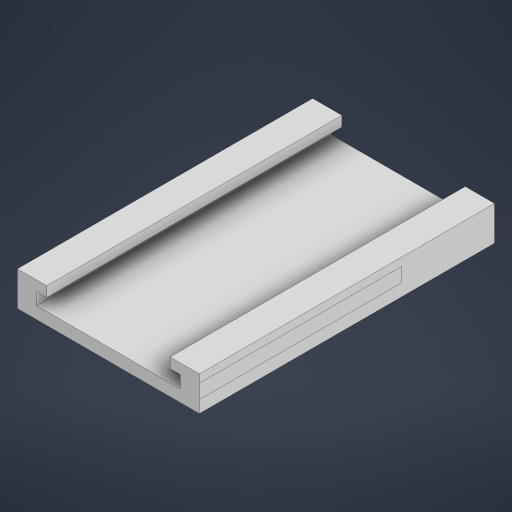
# Autodesk Inventor part: DINsupport
Saved by Autodesk Inventor 2023 (Build 270158000, 158)
## iProperties
Created: 2022-09-20
Part Number: DINsupport
Material: Generic
Document SubType Name: Modeling
Designer: CB110-09
Density: 1 g/cm^3
Appearance: Default
Author: CB110-09
Autodesk Inventor part; units mm, degrees
ref_plane "YZ Plane" through (0, 0, 0) normal (1, 0, 0) x (0, 1, 0)
ref_plane "XZ Plane" through (0, 0, 0) normal (0, 1, 0) x (-1, 0, 0)
ref_plane "XY Plane" through (0, 0, 0) normal (0, 0, 1) x (1, 0, 0)
sketch "Sketch1" plane through (0, 0, 0) normal (0, 1, 0) x (-1, 0, 0)
  line L0 (-32.5, 25) -> (32.5, 25)
  line L1 (32.5, 25) -> (32.5, -25)
  line L2 (32.5, -25) -> (-32.5, -25)
  line L3 (-32.5, -25) -> (-32.5, 25)
  line L4 (-32.5, 25) -> (32.5, -25) construction
  line L5 (32.5, 25) -> (-32.5, -25) construction
  point P0 (0, 0)
  dimension "d0" = 65
  dimension "d1" = 50
  constraints: 12 end point, 2 midpoint, 2 parallel, 1 horizontal, 1 perpendicular
  measures "d0" distance of L1.end L2.end
  measures "d1" distance of L0.end L1.end
extrude "Extrusion1" add sketch "Sketch1" along normal blind 3
sketch "Sketch2" plane through (0, 3, 0) normal (0, 1, 0) x (1, 0, 0)
  line L0 (32.5, 25) -> (-32.5, 25) projected
  line L1 (-18.25, -25) -> (18.25, -25)
  line L2 (18.25, -25) -> (18.25, 25)
  line L3 (18.25, 25) -> (-18.25, 25)
  line L4 (-18.25, 25) -> (-18.25, -25)
  line L5 (-18.25, -25) -> (18.25, 25) construction
  line L6 (18.25, -25) -> (-18.25, 25) construction
  line L7 (-22.5, -25) -> (22.5, -25)
  line L8 (22.5, -25) -> (22.5, 25)
  line L9 (22.5, 25) -> (-22.5, 25)
  line L10 (-22.5, 25) -> (-22.5, -25)
  line L11 (-22.5, -25) -> (22.5, 25) construction
  line L12 (22.5, -25) -> (-22.5, 25) construction
  point P0 (0, 0)
  dimension "d4" = 36.5
  dimension "d5" = 45
  constraints: 24 end point, 4 midpoint, 4 parallel, 2 horizontal, 2 perpendicular, 2 point on line
  measures "d4" distance of L3.end L2.end
  measures "d5" distance of L9.end L8.end
extrude "Extrusion2" add sketch "Sketch2" along normal blind 3.5 contours L8 L7 L2 L0 | L4 L7 L10 L0
sketch "Sketch3" plane through (0, 6.5, 0) normal (0, 1, 0) x (1, 0, 0)
  line L0 (-22.5, 25) -> (-32.5, 25) projected
  line L1 (-22.5, 25) -> (-15.25, 25)
  line L2 (-15.25, 25) -> (-15.25, -25)
  line L3 (-15.25, -25) -> (-22.5, -25)
  line L4 (-22.5, -25) -> (-22.5, 25)
  line L5 (-32.5, -25) -> (32.5, -25) projected
  line L6 (32.5, 25) -> (-32.5, 25) projected
  line L7 (22.4999, -25) -> (15.2499, -25)
  line L8 (15.2499, -25) -> (15.2499, 25)
  line L9 (15.2499, 25) -> (22.4999, 25)
  line L10 (22.4999, 25) -> (22.4999, -25)
  point P0 (0, 0)
  dimension "d8" = 7.25
  dimension "d9" = 7.25
  constraints: 16 end point, 4 parallel, 2 horizontal, 2 perpendicular, 2 point on line
  measures "d8" distance of L2.end L3.end
  measures "d9" distance of L8.end L9.end
extrude "Extrusion3" add sketch "Sketch3" along normal blind 2 contours L1 L2 L3 L4 | L6 L10 L5 L8
sketch "Sketch4" plane through (0, 3, 0) normal (0, 1, 0) x (1, 0, 0)
  line L0 (-22.5, 25) -> (-22.5, -25) projected
  line L1 (-32.5, 25) -> (-32.5, -25) projected
  line L2 (-22.5, 25) -> (-32.5, 25)
  line L3 (-32.5, 25) -> (-32.5, -25)
  line L4 (-32.5, -25) -> (-22.5, -25)
  line L5 (-22.5, -25) -> (-22.5, 25)
  line L6 (22.4999, -25) -> (22.4999, 25) projected
  line L7 (-32.5, -25) -> (32.5, -25) projected
  line L8 (22.4999, 25) -> (32.5, 25)
  line L9 (32.5, 25) -> (32.5, -25)
  line L10 (32.5, -25) -> (22.4999, -25)
  line L11 (22.4999, -25) -> (22.4999, 25)
  point P0 (0, 0)
  constraints: 16 end point, 4 parallel, 2 horizontal, 2 perpendicular
extrude "Extrusion4" cut sketch "Sketch4" against normal blind 10
sketch "Sketch5" plane through (-18.25, 3, 25) normal (1, 0, 0) x (0, 0, -1)
  line L0 (0, 3.5) -> (50, 3.5) projected
  line L1 (50, 0) -> (0, 0)
  line L2 (0, 0) -> (0, 3.5)
  line L3 (0, 3.5) -> (50, 3.5)
  line L4 (50, 3.5) -> (50, 0)
  point P0 (25, -3)
  constraints: 8 end point, 2 parallel, 1 horizontal, 1 perpendicular
extrude "Extrusion5" add sketch "Sketch5" along normal blind 0.5
sketch "Sketch6" plane through (18.25, 3, -25) normal (-1, 0, 0) x (0, 0, 1)
  line L0 (50, 0) -> (50, 3.5) projected
  line L1 (0, 0) -> (0, -3) projected
  line L2 (50, 3.5) -> (0, 3.5)
  line L3 (0, 3.5) -> (0, 0)
  line L4 (0, 0) -> (50, 0)
  line L5 (50, 0) -> (50, 3.5)
  point P0 (25, -3)
  constraints: 8 end point, 2 parallel, 1 horizontal, 1 perpendicular
extrude "Extrusion6" add sketch "Sketch6" along normal blind 0.5
sketch "Sketch7" plane through (0, 6.5, 0) normal (0, -1, 0) x (1, 0, 0)
  line L0 (15.2499, 25) -> (17.75, 25) projected
  line L1 (15.2499, -25) -> (17.75, -25)
  line L2 (17.75, -25) -> (17.75, 25)
  line L3 (17.75, 25) -> (15.2499, 25)
  line L4 (15.2499, 25) -> (15.2499, -25)
  line L5 (-15.25, 25) -> (-17.75, 25)
  line L6 (-17.75, 25) -> (-17.75, -25)
  line L7 (-17.75, -25) -> (-15.25, -25)
  line L8 (-15.25, -25) -> (-15.25, 25)
  point P0 (0, 0)
  constraints: 16 end point, 4 parallel, 2 horizontal, 2 perpendicular
extrude "Extrusion7" add sketch "Sketch7" along normal blind 0.5
sketch "Sketch8" plane through (-15.25, 8.5, -25) normal (0, 0, -1) x (-1, 0, 0)
  line L0 (0, -2.5) -> (0, 0) projected
  line L1 (0, -2.5) -> (0, 0)
  line L2 (7.25, 0) -> (0, 0) projected
  line L3 (0, 0) -> (7.25, 0)
  line L4 (7.25, 0) -> (7.25, -8.5) projected
  line L5 (7.25, 0) -> (7.25, -8.5)
  line L6 (7.25, -8.5) -> (-37.7499, -8.5) projected
  line L7 (7.25, -8.5) -> (-37.7499, -8.5)
  line L8 (-37.7499, -2) -> (-37.7499, 0) projected
  line L9 (-37.7499, -8.5) -> (-37.7499, 0)
  line L10 (-37.7499, 0) -> (-30.4999, 0) projected
  line L11 (-37.7499, 0) -> (-30.4999, 0)
  line L12 (-30.4999, -2.5) -> (-30.4999, 0) projected
  line L13 (-30.4999, 0) -> (-30.4999, -2.5)
  line L14 (-30.4999, -2.5) -> (-33, -2.5)
  line L15 (-33, -5.5) -> (-33, -2.5) projected
  line L16 (-33, -2.5) -> (-33, -5.5)
  line L17 (-33, -5.5) -> (2.5, -5.5) projected
  line L18 (-33, -5.5) -> (2.5, -5.5)
  line L19 (2.5, -2.5) -> (2.5, -5.5) projected
  line L20 (2.5, -5.5) -> (2.5, -2.5)
  line L21 (0, -2.5) -> (2.5, -2.5) projected
  line L22 (2.5, -2.5) -> (0, -2.5)
  point P0 (-15.25, -8.5)
  constraints: 24 end point, 7 perpendicular, 5 collinear
extrude "Extrusion8" add sketch "Sketch8" along normal blind 23
body "Solid1"
